Autodesk Fusion 360 part; units mm, degrees
(part 8 of 9)
  line L330 (-42.2083, 57.2942) -> (-37.8782, 54.7942)
  line L331 (-37.8782, 54.7942) -> (-33.5481, 57.2942)
  line L332 (-33.5481, 57.2942) -> (-33.5481, 62.2942)
  line L333 (-33.5481, 62.2942) -> (-37.8782, 64.7942)
  line L334 (-27.718, 64.7942) -> (-32.0481, 62.2942)
  line L335 (-32.0481, 62.2942) -> (-32.0481, 57.2942)
  line L336 (-32.0481, 57.2942) -> (-27.718, 54.7942)
  line L337 (-27.718, 54.7942) -> (-23.3878, 57.2942)
  line L338 (-23.3878, 57.2942) -> (-23.3878, 62.2942)
  line L339 (-23.3878, 62.2942) -> (-27.718, 64.7942)
  line L340 (-17.5577, 64.7942) -> (-21.8878, 62.2942)
  line L341 (-21.8878, 62.2942) -> (-21.8878, 57.2942)
  line L342 (-21.8878, 57.2942) -> (-17.5577, 54.7942)
  line L343 (-17.5577, 54.7942) -> (-13.2276, 57.2942)
  line L344 (-13.2276, 57.2942) -> (-13.2276, 62.2942)
  line L345 (-13.2276, 62.2942) -> (-17.5577, 64.7942)
  line L346 (-103.9199, 73.5933) -> (-108.25, 71.0933)
  line L347 (-108.25, 71.0933) -> (-108.25, 66.0933)
  line L348 (-108.25, 66.0933) -> (-103.9199, 63.5933)
  line L349 (-103.9199, 63.5933) -> (-99.5897, 66.0933)
  line L350 (-99.5897, 66.0933) -> (-99.5897, 71.0933)
  line L351 (-99.5897, 71.0933) -> (-103.9199, 73.5933)
  line L352 (-93.7596, 73.5933) -> (-98.0897, 71.0933)
  line L353 (-98.0897, 71.0933) -> (-98.0897, 66.0933)
  line L354 (-98.0897, 66.0933) -> (-93.7596, 63.5933)
  line L355 (-93.7596, 63.5933) -> (-89.4295, 66.0933)
  line L356 (-89.4295, 66.0933) -> (-89.4295, 71.0933)
  line L357 (-89.4295, 71.0933) -> (-93.7596, 73.5933)
  line L358 (-83.5994, 73.5933) -> (-87.9295, 71.0933)
  line L359 (-87.9295, 71.0933) -> (-87.9295, 66.0933)
  line L360 (-87.9295, 66.0933) -> (-83.5994, 63.5933)
  line L361 (-83.5994, 63.5933) -> (-79.2692, 66.0933)
  line L362 (-79.2692, 66.0933) -> (-79.2692, 71.0933)
  line L363 (-79.2692, 71.0933) -> (-83.5994, 73.5933)
  line L364 (-73.4391, 73.5933) -> (-77.7692, 71.0933)
  line L365 (-77.7692, 71.0933) -> (-77.7692, 66.0933)
  line L366 (-77.7692, 66.0933) -> (-73.4391, 63.5933)
  line L367 (-73.4391, 63.5933) -> (-69.109, 66.0933)
  line L368 (-69.109, 66.0933) -> (-69.109, 71.0933)
  line L369 (-69.109, 71.0933) -> (-73.4391, 73.5933)
  line L370 (-63.2789, 73.5933) -> (-67.609, 71.0933)
  line L371 (-67.609, 71.0933) -> (-67.609, 66.0933)
  line L372 (-67.609, 66.0933) -> (-63.2789, 63.5933)
  line L373 (-63.2789, 63.5933) -> (-58.9487, 66.0933)
  line L374 (-58.9487, 66.0933) -> (-58.9487, 71.0933)
  line L375 (-58.9487, 71.0933) -> (-63.2789, 73.5933)
  line L376 (-53.1186, 73.5933) -> (-57.4487, 71.0933)
  line L377 (-57.4487, 71.0933) -> (-57.4487, 66.0933)
  line L378 (-57.4487, 66.0933) -> (-53.1186, 63.5933)
  line L379 (-53.1186, 63.5933) -> (-48.7885, 66.0933)
  line L380 (-48.7885, 66.0933) -> (-48.7885, 71.0933)
  line L381 (-48.7885, 71.0933) -> (-53.1186, 73.5933)
  line L382 (-42.9583, 73.5933) -> (-47.2885, 71.0933)
  line L383 (-47.2885, 71.0933) -> (-47.2885, 66.0933)
  line L384 (-47.2885, 66.0933) -> (-42.9583, 63.5933)
  line L385 (-42.9583, 63.5933) -> (-38.6282, 66.0933)
  line L386 (-38.6282, 66.0933) -> (-38.6282, 71.0933)
  line L387 (-38.6282, 71.0933) -> (-42.9583, 73.5933)
  line L388 (-32.7981, 73.5933) -> (-37.1282, 71.0933)
  line L389 (-37.1282, 71.0933) -> (-37.1282, 66.0933)
  line L390 (-37.1282, 66.0933) -> (-32.7981, 63.5933)
  line L391 (-32.7981, 63.5933) -> (-28.468, 66.0933)
  line L392 (-28.468, 66.0933) -> (-28.468, 71.0933)
  line L393 (-28.468, 71.0933) -> (-32.7981, 73.5933)
  line L394 (-22.6378, 73.5933) -> (-26.968, 71.0933)
  line L395 (-26.968, 71.0933) -> (-26.968, 66.0933)
  line L396 (-26.968, 66.0933) -> (-22.6378, 63.5933)
  line L397 (-22.6378, 63.5933) -> (-18.3077, 66.0933)
  line L398 (-18.3077, 66.0933) -> (-18.3077, 71.0933)
  line L399 (-18.3077, 71.0933) -> (-22.6378, 73.5933)
  line L400 (-109, 82.3923) -> (-113.3301, 79.8923)
  line L401 (-113.3301, 79.8923) -> (-113.3301, 74.8923)
  line L402 (-113.3301, 74.8923) -> (-109, 72.3923)
  line L403 (-109, 72.3923) -> (-104.6699, 74.8923)
  line L404 (-104.6699, 74.8923) -> (-104.6699, 79.8923)
  line L405 (-104.6699, 79.8923) -> (-109, 82.3923)
  line L406 (-98.8397, 82.3923) -> (-103.1699, 79.8923)
  line L407 (-103.1699, 79.8923) -> (-103.1699, 74.8923)
  line L408 (-103.1699, 74.8923) -> (-98.8397, 72.3923)
  line L409 (-98.8397, 72.3923) -> (-94.5096, 74.8923)
  line L410 (-94.5096, 74.8923) -> (-94.5096, 79.8923)
  line L411 (-94.5096, 79.8923) -> (-98.8397, 82.3923)
  line L412 (-88.6795, 82.3923) -> (-93.0096, 79.8923)
  line L413 (-93.0096, 79.8923) -> (-93.0096, 74.8923)
  line L414 (-93.0096, 74.8923) -> (-88.6795, 72.3923)
  line L415 (-88.6795, 72.3923) -> (-84.3494, 74.8923)
  line L416 (-84.3494, 74.8923) -> (-84.3494, 79.8923)
  line L417 (-84.3494, 79.8923) -> (-88.6795, 82.3923)
  line L418 (-78.5192, 82.3923) -> (-82.8494, 79.8923)
  line L419 (-82.8494, 79.8923) -> (-82.8494, 74.8923)
  line L420 (-82.8494, 74.8923) -> (-78.5192, 72.3923)
  line L421 (-78.5192, 72.3923) -> (-74.1891, 74.8923)
  line L422 (-74.1891, 74.8923) -> (-74.1891, 79.8923)
  line L423 (-74.1891, 79.8923) -> (-78.5192, 82.3923)
  line L424 (-68.359, 82.3923) -> (-72.6891, 79.8923)
  line L425 (-72.6891, 79.8923) -> (-72.6891, 74.8923)
  line L426 (-72.6891, 74.8923) -> (-68.359, 72.3923)
  line L427 (-68.359, 72.3923) -> (-64.0289, 74.8923)
  line L428 (-64.0289, 74.8923) -> (-64.0289, 79.8923)
  line L429 (-64.0289, 79.8923) -> (-68.359, 82.3923)
  line L430 (-58.1987, 82.3923) -> (-62.5289, 79.8923)
  line L431 (-62.5289, 79.8923) -> (-62.5289, 74.8923)
  line L432 (-62.5289, 74.8923) -> (-58.1987, 72.3923)
  line L433 (-58.1987, 72.3923) -> (-53.8686, 74.8923)
  line L434 (-53.8686, 74.8923) -> (-53.8686, 79.8923)
  line L435 (-53.8686, 79.8923) -> (-58.1987, 82.3923)
  line L436 (-48.0385, 82.3923) -> (-52.3686, 79.8923)
  line L437 (-52.3686, 79.8923) -> (-52.3686, 74.8923)
  line L438 (-52.3686, 74.8923) -> (-48.0385, 72.3923)
  line L439 (-48.0385, 72.3923) -> (-43.7083, 74.8923)
  line L440 (-43.7083, 74.8923) -> (-43.7083, 79.8923)
  line L441 (-43.7083, 79.8923) -> (-48.0385, 82.3923)
  line L442 (-37.8782, 82.3923) -> (-42.2083, 79.8923)
  line L443 (-42.2083, 79.8923) -> (-42.2083, 74.8923)
  line L444 (-42.2083, 74.8923) -> (-37.8782, 72.3923)
  line L445 (-37.8782, 72.3923) -> (-33.5481, 74.8923)
  line L446 (-33.5481, 74.8923) -> (-33.5481, 79.8923)
  line L447 (-33.5481, 79.8923) -> (-37.8782, 82.3923)
  line L448 (-27.718, 82.3923) -> (-32.0481, 79.8923)
  line L449 (-32.0481, 79.8923) -> (-32.0481, 74.8923)
  line L450 (-32.0481, 74.8923) -> (-27.718, 72.3923)
  line L451 (-27.718, 72.3923) -> (-23.3878, 74.8923)
  line L452 (-23.3878, 74.8923) -> (-23.3878, 79.8923)
  line L453 (-23.3878, 79.8923) -> (-27.718, 82.3923)
  line L454 (-17.5577, 82.3923) -> (-21.8878, 79.8923)
  line L455 (-21.8878, 79.8923) -> (-21.8878, 74.8923)
  line L456 (-21.8878, 74.8923) -> (-17.5577, 72.3923)
  line L457 (-17.5577, 72.3923) -> (-13.2276, 74.8923)
  line L458 (-13.2276, 74.8923) -> (-13.2276, 79.8923)
  line L459 (-13.2276, 79.8923) -> (-17.5577, 82.3923)
  line L460 (-103.9199, 91.1913) -> (-108.25, 88.6913)
  line L461 (-108.25, 88.6913) -> (-108.25, 83.6913)
  line L462 (-108.25, 83.6913) -> (-103.9199, 81.1913)
  line L463 (-103.9199, 81.1913) -> (-99.5897, 83.6913)
  line L464 (-99.5897, 83.6913) -> (-99.5897, 88.6913)
  line L465 (-99.5897, 88.6913) -> (-103.9199, 91.1913)
  line L466 (-93.7596, 91.1913) -> (-98.0897, 88.6913)
  line L467 (-98.0897, 88.6913) -> (-98.0897, 83.6913)
  line L468 (-98.0897, 83.6913) -> (-93.7596, 81.1913)
  line L469 (-93.7596, 81.1913) -> (-89.4295, 83.6913)
  line L470 (-89.4295, 83.6913) -> (-89.4295, 88.6913)
  line L471 (-89.4295, 88.6913) -> (-93.7596, 91.1913)
  line L472 (-83.5994, 91.1913) -> (-87.9295, 88.6913)
  line L473 (-87.9295, 88.6913) -> (-87.9295, 83.6913)
  line L474 (-87.9295, 83.6913) -> (-83.5994, 81.1913)
  line L475 (-83.5994, 81.1913) -> (-79.2692, 83.6913)
  line L476 (-79.2692, 83.6913) -> (-79.2692, 88.6913)
  line L477 (-79.2692, 88.6913) -> (-83.5994, 91.1913)
  line L478 (-73.4391, 91.1913) -> (-77.7692, 88.6913)
  line L479 (-77.7692, 88.6913) -> (-77.7692, 83.6913)
  line L480 (-77.7692, 83.6913) -> (-73.4391, 81.1913)
  line L481 (-73.4391, 81.1913) -> (-69.109, 83.6913)
  line L482 (-69.109, 83.6913) -> (-69.109, 88.6913)
  line L483 (-69.109, 88.6913) -> (-73.4391, 91.1913)
  line L484 (-63.2789, 91.1913) -> (-67.609, 88.6913)
  line L485 (-67.609, 88.6913) -> (-67.609, 83.6913)
  line L486 (-67.609, 83.6913) -> (-63.2789, 81.1913)
  line L487 (-63.2789, 81.1913) -> (-58.9487, 83.6913)
  line L488 (-58.9487, 83.6913) -> (-58.9487, 88.6913)
  line L489 (-58.9487, 88.6913) -> (-63.2789, 91.1913)
  line L490 (-53.1186, 91.1913) -> (-57.4487, 88.6913)
  line L491 (-57.4487, 88.6913) -> (-57.4487, 83.6913)
  line L492 (-57.4487, 83.6913) -> (-53.1186, 81.1913)
  line L493 (-53.1186, 81.1913) -> (-48.7885, 83.6913)
  line L494 (-48.7885, 83.6913) -> (-48.7885, 88.6913)
  line L495 (-48.7885, 88.6913) -> (-53.1186, 91.1913)
  line L496 (-42.9583, 91.1913) -> (-47.2885, 88.6913)
  line L497 (-47.2885, 88.6913) -> (-47.2885, 83.6913)
  line L498 (-47.2885, 83.6913) -> (-42.9583, 81.1913)
  line L499 (-42.9583, 81.1913) -> (-38.6282, 83.6913)
  line L500 (-38.6282, 83.6913) -> (-38.6282, 88.6913)
  line L501 (-38.6282, 88.6913) -> (-42.9583, 91.1913)
  line L502 (-32.7981, 91.1913) -> (-37.1282, 88.6913)
  line L503 (-37.1282, 88.6913) -> (-37.1282, 83.6913)
  line L504 (-37.1282, 83.6913) -> (-32.7981, 81.1913)
  line L505 (-32.7981, 81.1913) -> (-28.468, 83.6913)
  line L506 (-28.468, 83.6913) -> (-28.468, 88.6913)
  line L507 (-28.468, 88.6913) -> (-32.7981, 91.1913)
  line L508 (-22.6378, 91.1913) -> (-26.968, 88.6913)
  line L509 (-26.968, 88.6913) -> (-26.968, 83.6913)
  line L510 (-26.968, 83.6913) -> (-22.6378, 81.1913)
  line L511 (-22.6378, 81.1913) -> (-18.3077, 83.6913)
  line L512 (-18.3077, 83.6913) -> (-18.3077, 88.6913)
  line L513 (-18.3077, 88.6913) -> (-22.6378, 91.1913)
  line L514 (-109, 99.9904) -> (-113.3301, 97.4904)
  line L515 (-113.3301, 97.4904) -> (-113.3301, 92.4904)
  line L516 (-113.3301, 92.4904) -> (-109, 89.9904)
  line L517 (-109, 89.9904) -> (-104.6699, 92.4904)
  line L518 (-104.6699, 92.4904) -> (-104.6699, 97.4904)
  line L519 (-104.6699, 97.4904) -> (-109, 99.9904)
  line L520 (-98.8397, 99.9904) -> (-103.1699, 97.4904)
  line L521 (-103.1699, 97.4904) -> (-103.1699, 92.4904)
  line L522 (-103.1699, 92.4904) -> (-98.8397, 89.9904)
  line L523 (-98.8397, 89.9904) -> (-94.5096, 92.4904)
  line L524 (-94.5096, 92.4904) -> (-94.5096, 97.4904)
  line L525 (-94.5096, 97.4904) -> (-98.8397, 99.9904)
  line L526 (-88.6795, 99.9904) -> (-93.0096, 97.4904)
  line L527 (-93.0096, 97.4904) -> (-93.0096, 92.4904)
  line L528 (-93.0096, 92.4904) -> (-88.6795, 89.9904)
  line L529 (-88.6795, 89.9904) -> (-84.3494, 92.4904)
  line L530 (-84.3494, 92.4904) -> (-84.3494, 97.4904)
  line L531 (-84.3494, 97.4904) -> (-88.6795, 99.9904)
  line L532 (-78.5192, 99.9904) -> (-82.8494, 97.4904)
  line L533 (-82.8494, 97.4904) -> (-82.8494, 92.4904)
  line L534 (-82.8494, 92.4904) -> (-78.5192, 89.9904)
  line L535 (-78.5192, 89.9904) -> (-74.1891, 92.4904)
  line L536 (-74.1891, 92.4904) -> (-74.1891, 97.4904)
  line L537 (-74.1891, 97.4904) -> (-78.5192, 99.9904)
  line L538 (-68.359, 99.9904) -> (-72.6891, 97.4904)
  line L539 (-72.6891, 97.4904) -> (-72.6891, 92.4904)
  line L540 (-72.6891, 92.4904) -> (-68.359, 89.9904)
  line L541 (-68.359, 89.9904) -> (-64.0289, 92.4904)
  line L542 (-64.0289, 92.4904) -> (-64.0289, 97.4904)
  line L543 (-64.0289, 97.4904) -> (-68.359, 99.9904)
  line L544 (-58.1987, 99.9904) -> (-62.5289, 97.4904)
  line L545 (-62.5289, 97.4904) -> (-62.5289, 92.4904)
  line L546 (-62.5289, 92.4904) -> (-58.1987, 89.9904)
  line L547 (-58.1987, 89.9904) -> (-53.8686, 92.4904)
  line L548 (-53.8686, 92.4904) -> (-53.8686, 97.4904)
  line L549 (-53.8686, 97.4904) -> (-58.1987, 99.9904)
  line L550 (-48.0385, 99.9904) -> (-52.3686, 97.4904)
  line L551 (-52.3686, 97.4904) -> (-52.3686, 92.4904)
  line L552 (-52.3686, 92.4904) -> (-48.0385, 89.9904)
  line L553 (-48.0385, 89.9904) -> (-43.7083, 92.4904)
  line L554 (-43.7083, 92.4904) -> (-43.7083, 97.4904)
  line L555 (-43.7083, 97.4904) -> (-48.0385, 99.9904)
  line L556 (-37.8782, 99.9904) -> (-42.2083, 97.4904)
  line L557 (-42.2083, 97.4904) -> (-42.2083, 92.4904)
  line L558 (-42.2083, 92.4904) -> (-37.8782, 89.9904)
  line L559 (-37.8782, 89.9904) -> (-33.5481, 92.4904)
  line L560 (-33.5481, 92.4904) -> (-33.5481, 97.4904)
  line L561 (-33.5481, 97.4904) -> (-37.8782, 99.9904)
  line L562 (-27.718, 99.9904) -> (-32.0481, 97.4904)
  line L563 (-32.0481, 97.4904) -> (-32.0481, 92.4904)
  line L564 (-32.0481, 92.4904) -> (-27.718, 89.9904)
  line L565 (-27.718, 89.9904) -> (-23.3878, 92.4904)
  line L566 (-23.3878, 92.4904) -> (-23.3878, 97.4904)
  line L567 (-23.3878, 97.4904) -> (-27.718, 99.9904)
  line L568 (-17.5577, 99.9904) -> (-21.8878, 97.4904)
  line L569 (-21.8878, 97.4904) -> (-21.8878, 92.4904)
  line L570 (-21.8878, 92.4904) -> (-17.5577, 89.9904)
  line L571 (-17.5577, 89.9904) -> (-13.2276, 92.4904)
  line L572 (-13.2276, 92.4904) -> (-13.2276, 97.4904)
  line L573 (-13.2276, 97.4904) -> (-17.5577, 99.9904)
  line L574 (-103.9199, 108.7894) -> (-108.25, 106.2894)
  line L575 (-108.25, 106.2894) -> (-108.25, 101.2894)
  line L576 (-108.25, 101.2894) -> (-103.9199, 98.7894)
  line L577 (-103.9199, 98.7894) -> (-99.5897, 101.2894)
  line L578 (-99.5897, 101.2894) -> (-99.5897, 106.2894)
  line L579 (-99.5897, 106.2894) -> (-103.9199, 108.7894)
  line L580 (-93.7596, 108.7894) -> (-98.0897, 106.2894)
  line L581 (-98.0897, 106.2894) -> (-98.0897, 101.2894)
  line L582 (-98.0897, 101.2894) -> (-93.7596, 98.7894)
  line L583 (-93.7596, 98.7894) -> (-89.4295, 101.2894)
  line L584 (-89.4295, 101.2894) -> (-89.4295, 106.2894)
  line L585 (-89.4295, 106.2894) -> (-93.7596, 108.7894)
  line L586 (-83.5994, 108.7894) -> (-87.9295, 106.2894)
  line L587 (-87.9295, 106.2894) -> (-87.9295, 101.2894)
  line L588 (-87.9295, 101.2894) -> (-83.5994, 98.7894)
  line L589 (-83.5994, 98.7894) -> (-79.2692, 101.2894)
  line L590 (-79.2692, 101.2894) -> (-79.2692, 106.2894)
  line L591 (-79.2692, 106.2894) -> (-83.5994, 108.7894)
  line L592 (-73.4391, 108.7894) -> (-77.7692, 106.2894)
  line L593 (-77.7692, 106.2894) -> (-77.7692, 101.2894)
  line L594 (-77.7692, 101.2894) -> (-73.4391, 98.7894)
  line L595 (-73.4391, 98.7894) -> (-69.109, 101.2894)
  line L596 (-69.109, 101.2894) -> (-69.109, 106.2894)
  line L597 (-69.109, 106.2894) -> (-73.4391, 108.7894)
  line L598 (-63.2789, 108.7894) -> (-67.609, 106.2894)
  line L599 (-67.609, 106.2894) -> (-67.609, 101.2894)
  line L600 (-67.609, 101.2894) -> (-63.2789, 98.7894)
  line L601 (-63.2789, 98.7894) -> (-58.9487, 101.2894)
  line L602 (-58.9487, 101.2894) -> (-58.9487, 106.2894)
  line L603 (-58.9487, 106.2894) -> (-63.2789, 108.7894)
  line L604 (-53.1186, 108.7894) -> (-57.4487, 106.2894)
  line L605 (-57.4487, 106.2894) -> (-57.4487, 101.2894)
  line L606 (-57.4487, 101.2894) -> (-53.1186, 98.7894)
  line L607 (-53.1186, 98.7894) -> (-48.7885, 101.2894)
  line L608 (-48.7885, 101.2894) -> (-48.7885, 106.2894)
  line L609 (-48.7885, 106.2894) -> (-53.1186, 108.7894)
  line L610 (-42.9583, 108.7894) -> (-47.2885, 106.2894)
  line L611 (-47.2885, 106.2894) -> (-47.2885, 101.2894)
  line L612 (-47.2885, 101.2894) -> (-42.9583, 98.7894)
  line L613 (-42.9583, 98.7894) -> (-38.6282, 101.2894)
  line L614 (-38.6282, 101.2894) -> (-38.6282, 106.2894)
  line L615 (-38.6282, 106.2894) -> (-42.9583, 108.7894)
  line L616 (-32.7981, 108.7894) -> (-37.1282, 106.2894)
  line L617 (-37.1282, 106.2894) -> (-37.1282, 101.2894)
  line L618 (-37.1282, 101.2894) -> (-32.7981, 98.7894)
  line L619 (-32.7981, 98.7894) -> (-28.468, 101.2894)
  line L620 (-28.468, 101.2894) -> (-28.468, 106.2894)
  line L621 (-28.468, 106.2894) -> (-32.7981, 108.7894)
  line L622 (-22.6378, 108.7894) -> (-26.968, 106.2894)
  line L623 (-26.968, 106.2894) -> (-26.968, 101.2894)
  line L624 (-26.968, 101.2894) -> (-22.6378, 98.7894)
  line L625 (-22.6378, 98.7894) -> (-18.3077, 101.2894)
  line L626 (-18.3077, 101.2894) -> (-18.3077, 106.2894)
  line L627 (-18.3077, 106.2894) -> (-22.6378, 108.7894)
  line L628 (-109, 117.5885) -> (-113.3301, 115.0885)
  line L629 (-113.3301, 115.0885) -> (-113.3301, 110.0885)
  line L630 (-113.3301, 110.0885) -> (-109, 107.5885)
  line L631 (-109, 107.5885) -> (-104.6699, 110.0885)
  line L632 (-104.6699, 110.0885) -> (-104.6699, 115.0885)
  line L633 (-104.6699, 115.0885) -> (-109, 117.5885)
  line L634 (-98.8397, 117.5885) -> (-103.1699, 115.0885)
  line L635 (-103.1699, 115.0885) -> (-103.1699, 110.0885)
  line L636 (-103.1699, 110.0885) -> (-98.8397, 107.5885)
  line L637 (-98.8397, 107.5885) -> (-94.5096, 110.0885)
  line L638 (-94.5096, 110.0885) -> (-94.5096, 115.0885)
  line L639 (-94.5096, 115.0885) -> (-98.8397, 117.5885)
  line L640 (-88.6795, 117.5885) -> (-93.0096, 115.0885)
  line L641 (-93.0096, 115.0885) -> (-93.0096, 110.0885)
  line L642 (-93.0096, 110.0885) -> (-88.6795, 107.5885)
  line L643 (-88.6795, 107.5885) -> (-84.3494, 110.0885)
  line L644 (-84.3494, 110.0885) -> (-84.3494, 115.0885)
  line L645 (-84.3494, 115.0885) -> (-88.6795, 117.5885)
  line L646 (-78.5192, 117.5885) -> (-82.8494, 115.0885)
  line L647 (-82.8494, 115.0885) -> (-82.8494, 110.0885)
  line L648 (-82.8494, 110.0885) -> (-78.5192, 107.5885)
  line L649 (-78.5192, 107.5885) -> (-74.1891, 110.0885)
  line L650 (-74.1891, 110.0885) -> (-74.1891, 115.0885)
  line L651 (-74.1891, 115.0885) -> (-78.5192, 117.5885)
  line L652 (-68.359, 117.5885) -> (-72.6891, 115.0885)
  line L653 (-72.6891, 115.0885) -> (-72.6891, 110.0885)
  line L654 (-72.6891, 110.0885) -> (-68.359, 107.5885)
  line L655 (-68.359, 107.5885) -> (-64.0289, 110.0885)
  line L656 (-64.0289, 110.0885) -> (-64.0289, 115.0885)
  line L657 (-64.0289, 115.0885) -> (-68.359, 117.5885)
  line L658 (-58.1987, 117.5885) -> (-62.5289, 115.0885)
  line L659 (-62.5289, 115.0885) -> (-62.5289, 110.0885)
  line L660 (-62.5289, 110.0885) -> (-58.1987, 107.5885)
  line L661 (-58.1987, 107.5885) -> (-53.8686, 110.0885)
  line L662 (-53.8686, 110.0885) -> (-53.8686, 115.0885)
  line L663 (-53.8686, 115.0885) -> (-58.1987, 117.5885)
  line L664 (-48.0385, 117.5885) -> (-52.3686, 115.0885)
  line L665 (-52.3686, 115.0885) -> (-52.3686, 110.0885)
  line L666 (-52.3686, 110.0885) -> (-48.0385, 107.5885)
  line L667 (-48.0385, 107.5885) -> (-43.7083, 110.0885)
  line L668 (-43.7083, 110.0885) -> (-43.7083, 115.0885)
  line L669 (-43.7083, 115.0885) -> (-48.0385, 117.5885)
  line L670 (-37.8782, 117.5885) -> (-42.2083, 115.0885)
  line L671 (-42.2083, 115.0885) -> (-42.2083, 110.0885)
  line L672 (-42.2083, 110.0885) -> (-37.8782, 107.5885)
  line L673 (-37.8782, 107.5885) -> (-33.5481, 110.0885)
  line L674 (-33.5481, 110.0885) -> (-33.5481, 115.0885)
  line L675 (-33.5481, 115.0885) -> (-37.8782, 117.5885)
  line L676 (-27.718, 117.5885) -> (-32.0481, 115.0885)
  line L677 (-32.0481, 115.0885) -> (-32.0481, 110.0885)
  line L678 (-32.0481, 110.0885) -> (-27.718, 107.5885)
  line L679 (-27.718, 107.5885) -> (-23.3878, 110.0885)
  line L680 (-23.3878, 110.0885) -> (-23.3878, 115.0885)
  line L681 (-23.3878, 115.0885) -> (-27.718, 117.5885)
  line L682 (-17.5577, 117.5885) -> (-21.8878, 115.0885)
  line L683 (-21.8878, 115.0885) -> (-21.8878, 110.0885)
  line L684 (-21.8878, 110.0885) -> (-17.5577, 107.5885)
  line L685 (-17.5577, 107.5885) -> (-13.2276, 110.0885)
  line L686 (-13.2276, 110.0885) -> (-13.2276, 115.0885)
  line L687 (-13.2276, 115.0885) -> (-17.5577, 117.5885)
extrude "拉伸26" cut sketch "草图26" against normal blind 5 contours L4 L5 L6 L7 L8 L9 | L10 L11 L12 L13 L14 L15 | L16 L17 L18 L19 L20 L21 | L22 L23 L24 L25 L26 L27 | L28 L29 L30 L31 L32 L33 | L34 L35 L36 L37 L38 L39 | L40 L41 L42 L43 L44 L45 | L46 L47 L48 L49 L50 L51 | L52 L53 L54 L55 L56 L57 | L58 L59 L60 L61 L62 L63 | L64 L65 L66 L67 L68 L69 | L70 L71 L72 L73 L74 L75 | L76 L77 L78 L79 L80 L81 | L82 L83 L84 L85 L86 L87 | L88 L89 L90 L91 L92 L93 | L94 L95 L96 L97 L98 L99 | L100 L101 L102 L103 L104 L105 | L106 L107 L108 L109 L110 L111 | L112 L113 L114 L115 L116 L117 | L118 L119 L120 L121 L122 L123 | L124 L125 L126 L127 L128 L129 | L130 L131 L132 L133 L134 L135 | L136 L137 L138 L139 L140 L141 | L142 L143 L144 L145 L146 L147 | L148 L149 L150 L151 L152 L153 | L154 L155 L156 L157 L158 L159 | L160 L161 L162 L163 L164 L165 | L166 L167 L168 L169 L170 L171 | L172 L173 L174 L175 L176 L177 | L178 L179 L180 L181 L182 L183 | L184 L185 L186 L187 L188 L189 | L190 L191 L192 L193 L194 L195 | L196 L197 L198 L199 L200 L201 | L202 L203 L204 L205 L206 L207 | L208 L209 L210 L211 L212 L213 | L214 L215 L216 L217 L218 L219 | L220 L221 L222 L223 L224 L225 | L226 L227 L228 L229 L230 L231 | L232 L233 L234 L235 L236 L237 | L238 L239 L240 L241 L242 L243 | L244 L245 L246 L247 L248 L249 | L250 L251 L252 L253 L254 L255 | L256 L257 L258 L259 L260 L261 | L262 L263 L264 L265 L266 L267 | L268 L269 L270 L271 L272 L273 | L274 L275 L276 L277 L278 L279 | L280 L281 L282 L283 L284 L285 | L286 L287 L288 L289 L290 L291 | L292 L293 L294 L295 L296 L297 | L298 L299 L300 L301 L302 L303 | L304 L305 L306 L307 L308 L309 | L310 L311 L312 L313 L314 L315 | L316 L317 L318 L319 L320 L321 | L322 L323 L324 L325 L326 L327 | L328 L329 L330 L331 L332 L333 | L334 L335 L336 L337 L338 L339 | L340 L341 L342 L343 L344 L345 | L346 L347 L348 L349 L350 L351 | L352 L353 L354 L355 L356 L357 | L358 L359 L360 L361 L362 L363 | L364 L365 L366 L367 L368 L369 | L370 L371 L372 L373 L374 L375 | L376 L377 L378 L379 L380 L381 | L382 L383 L384 L385 L386 L387 | L388 L389 L390 L391 L392 L393 | L394 L395 L396 L397 L398 L399 | L400 L401 L402 L403 L404 L405 | L406 L407 L408 L409 L410 L411 | L412 L413 L414 L415 L416 L417 | L418 L419 L420 L421 L422 L423 | L424 L425 L426 L427 L428 L429 | L430 L431 L432 L433 L434 L435 | L436 L437 L438 L439 L440 L441 | L442 L443 L444 L445 L446 L447 | L448 L449 L450 L451 L452 L453 | L454 L455 L456 L457 L458 L459 | L460 L461 L462 L463 L464 L465 | L466 L467 L468 L469 L470 L471 | L472 L473 L474 L475 L476 L477 | L478 L479 L480 L481 L482 L483 | L484 L485 L486 L487 L488 L489 | L490 L491 L492 L493 L494 L495 | L496 L497 L498 L499 L500 L501 | L502 L503 L504 L505 L506 L507 | L508 L509 L510 L511 L512 L513 | L514 L515 L516 L517 L518 L519 | L520 L521 L522 L523 L524 L525 | L526 L527 L528 L529 L530 L531 | L532 L533 L534 L535 L536 L537 | L538 L539 L540 L541 L542 L543 | L544 L545 L546 L547 L548 L549 | L550 L551 L552 L553 L554 L555 | L556 L557 L558 L559 L560 L561 | L562 L563 L564 L565 L566 L567 | L568 L569 L570 L571 L572 L573 | L574 L575 L576 L577 L578 L579 | L580 L581 L582 L583 L584 L585 | L586 L587 L588 L589 L590 L591 | L592 L593 L594 L595 L596 L597 | L598 L599 L600 L601 L602 L603 | L604 L605 L606 L607 L608 L609 | L610 L611 L612 L613 L614 L615 | L616 L617 L618 L619 L620 L621 | L622 L623 L624 L625 L626 L627 | L628 L629 L630 L631 L632 L633 | L634 L635 L636 L637 L638 L639 | L640 L641 L642 L643 L644 L645 | L646 L647 L648 L649 L650 L651 | L652 L653 L654 L655 L656 L657 | L658 L659 L660 L661 L662 L663 | L664 L665 L666 L667 L668 L669 | L670 L671 L672 L673 L674 L675 | L676 L677 L678 L679 L680 L681 | L682 L683 L684 L685 L686 L687 bodies 1 4
sketch "草图27" plane through (116, 0, 0) normal (-1, 0, 0) x (0, -1, 0)
  line L0 (7, 0) -> (116, 0)
  line L1 (116, 0) -> (116, 120)
  line L2 (116, 120) -> (7, 120)
  line L3 (7, 120) -> (7, 0)
  line L4 (19.0801, 20.799) -> (14.75, 18.299)
  line L5 (14.75, 18.299) -> (14.75, 13.299)
  line L6 (14.75, 13.299) -> (19.0801, 10.799)
  line L7 (19.0801, 10.799) -> (23.4103, 13.299)
  line L8 (23.4103, 13.299) -> (23.4103, 18.299)
  line L9 (23.4103, 18.299) -> (19.0801, 20.799)
  line L10 (29.2404, 20.799) -> (24.9103, 18.299)
  line L11 (24.9103, 18.299) -> (24.9103, 13.299)
  line L12 (24.9103, 13.299) -> (29.2404, 10.799)
  line L13 (29.2404, 10.799) -> (33.5705, 13.299)
  line L14 (33.5705, 13.299) -> (33.5705, 18.299)
  line L15 (33.5705, 18.299) -> (29.2404, 20.799)
  line L16 (39.4006, 20.799) -> (35.0705, 18.299)
  line L17 (35.0705, 18.299) -> (35.0705, 13.299)
  line L18 (35.0705, 13.299) -> (39.4006, 10.799)
  line L19 (39.4006, 10.799) -> (43.7308, 13.299)
  line L20 (43.7308, 13.299) -> (43.7308, 18.299)
  line L21 (43.7308, 18.299) -> (39.4006, 20.799)
  line L22 (49.5609, 20.799) -> (45.2308, 18.299)
  line L23 (45.2308, 18.299) -> (45.2308, 13.299)
  line L24 (45.2308, 13.299) -> (49.5609, 10.799)
  line L25 (49.5609, 10.799) -> (53.891, 13.299)
  line L26 (53.891, 13.299) -> (53.891, 18.299)
  line L27 (53.891, 18.299) -> (49.5609, 20.799)
  line L28 (59.7211, 20.799) -> (55.391, 18.299)
  line L29 (55.391, 18.299) -> (55.391, 13.299)
  line L30 (55.391, 13.299) -> (59.7211, 10.799)
  line L31 (59.7211, 10.799) -> (64.0513, 13.299)
  line L32 (64.0513, 13.299) -> (64.0513, 18.299)
  line L33 (64.0513, 18.299) -> (59.7211, 20.799)
  line L34 (69.8814, 20.799) -> (65.5513, 18.299)
  line L35 (65.5513, 18.299) -> (65.5513, 13.299)
  line L36 (65.5513, 13.299) -> (69.8814, 10.799)
  line L37 (69.8814, 10.799) -> (74.2115, 13.299)
  line L38 (74.2115, 13.299) -> (74.2115, 18.299)
  line L39 (74.2115, 18.299) -> (69.8814, 20.799)
  line L40 (80.0416, 20.799) -> (75.7115, 18.299)
  line L41 (75.7115, 18.299) -> (75.7115, 13.299)
  line L42 (75.7115, 13.299) -> (80.0416, 10.799)
  line L43 (80.0416, 10.799) -> (84.3718, 13.299)
  line L44 (84.3718, 13.299) -> (84.3718, 18.299)
  line L45 (84.3718, 18.299) -> (80.0416, 20.799)
  line L46 (90.2019, 20.799) -> (85.8718, 18.299)
  line L47 (85.8718, 18.299) -> (85.8718, 13.299)
  line L48 (85.8718, 13.299) -> (90.2019, 10.799)
  line L49 (90.2019, 10.799) -> (94.532, 13.299)
  line L50 (94.532, 13.299) -> (94.532, 18.299)
  line L51 (94.532, 18.299) -> (90.2019, 20.799)
  line L52 (100.3622, 20.799) -> (96.032, 18.299)
  line L53 (96.032, 18.299) -> (96.032, 13.299)
  line L54 (96.032, 13.299) -> (100.3622, 10.799)
  line L55 (100.3622, 10.799) -> (104.6923, 13.299)
  line L56 (104.6923, 13.299) -> (104.6923, 18.299)
  line L57 (104.6923, 18.299) -> (100.3622, 20.799)
  line L58 (14, 29.5981) -> (9.6699, 27.0981)
  line L59 (9.6699, 27.0981) -> (9.6699, 22.0981)
  line L60 (9.6699, 22.0981) -> (14, 19.5981)
  line L61 (14, 19.5981) -> (18.3301, 22.0981)
  line L62 (18.3301, 22.0981) -> (18.3301, 27.0981)
  line L63 (18.3301, 27.0981) -> (14, 29.5981)
  line L64 (24.1603, 29.5981) -> (19.8301, 27.0981)
  line L65 (19.8301, 27.0981) -> (19.8301, 22.0981)
  line L66 (19.8301, 22.0981) -> (24.1603, 19.5981)
  line L67 (24.1603, 19.5981) -> (28.4904, 22.0981)
  line L68 (28.4904, 22.0981) -> (28.4904, 27.0981)
  line L69 (28.4904, 27.0981) -> (24.1603, 29.5981)
  line L70 (34.3205, 29.5981) -> (29.9904, 27.0981)
  line L71 (29.9904, 27.0981) -> (29.9904, 22.0981)
  line L72 (29.9904, 22.0981) -> (34.3205, 19.5981)
  line L73 (34.3205, 19.5981) -> (38.6506, 22.0981)
  line L74 (38.6506, 22.0981) -> (38.6506, 27.0981)
  line L75 (38.6506, 27.0981) -> (34.3205, 29.5981)
  line L76 (44.4808, 29.5981) -> (40.1506, 27.0981)
  line L77 (40.1506, 27.0981) -> (40.1506, 22.0981)
  line L78 (40.1506, 22.0981) -> (44.4808, 19.5981)
  line L79 (44.4808, 19.5981) -> (48.8109, 22.0981)
  line L80 (48.8109, 22.0981) -> (48.8109, 27.0981)
  line L81 (48.8109, 27.0981) -> (44.4808, 29.5981)
  line L82 (54.641, 29.5981) -> (50.3109, 27.0981)
  line L83 (50.3109, 27.0981) -> (50.3109, 22.0981)
  line L84 (50.3109, 22.0981) -> (54.641, 19.5981)
  line L85 (54.641, 19.5981) -> (58.9711, 22.0981)
  line L86 (58.9711, 22.0981) -> (58.9711, 27.0981)
  line L87 (58.9711, 27.0981) -> (54.641, 29.5981)
  line L88 (64.8013, 29.5981) -> (60.4711, 27.0981)
  line L89 (60.4711, 27.0981) -> (60.4711, 22.0981)
  line L90 (60.4711, 22.0981) -> (64.8013, 19.5981)
  line L91 (64.8013, 19.5981) -> (69.1314, 22.0981)
  line L92 (69.1314, 22.0981) -> (69.1314, 27.0981)
  line L93 (69.1314, 27.0981) -> (64.8013, 29.5981)
  line L94 (74.9615, 29.5981) -> (70.6314, 27.0981)
  line L95 (70.6314, 27.0981) -> (70.6314, 22.0981)
  line L96 (70.6314, 22.0981) -> (74.9615, 19.5981)
  line L97 (74.9615, 19.5981) -> (79.2916, 22.0981)
  line L98 (79.2916, 22.0981) -> (79.2916, 27.0981)
  line L99 (79.2916, 27.0981) -> (74.9615, 29.5981)
  line L100 (85.1218, 29.5981) -> (80.7916, 27.0981)
  line L101 (80.7916, 27.0981) -> (80.7916, 22.0981)
  line L102 (80.7916, 22.0981) -> (85.1218, 19.5981)
  line L103 (85.1218, 19.5981) -> (89.4519, 22.0981)
  line L104 (89.4519, 22.0981) -> (89.4519, 27.0981)
  line L105 (89.4519, 27.0981) -> (85.1218, 29.5981)
  line L106 (95.282, 29.5981) -> (90.9519, 27.0981)
  line L107 (90.9519, 27.0981) -> (90.9519, 22.0981)
  line L108 (90.9519, 22.0981) -> (95.282, 19.5981)
  line L109 (95.282, 19.5981) -> (99.6122, 22.0981)
  line L110 (99.6122, 22.0981) -> (99.6122, 27.0981)
  line L111 (99.6122, 27.0981) -> (95.282, 29.5981)
  line L112 (105.4423, 29.5981) -> (101.1122, 27.0981)
  line L113 (101.1122, 27.0981) -> (101.1122, 22.0981)
  line L114 (101.1122, 22.0981) -> (105.4423, 19.5981)
  line L115 (105.4423, 19.5981) -> (109.7724, 22.0981)
  line L116 (109.7724, 22.0981) -> (109.7724, 27.0981)
  line L117 (109.7724, 27.0981) -> (105.4423, 29.5981)
  line L118 (19.0801, 38.3971) -> (14.75, 35.8971)
  line L119 (14.75, 35.8971) -> (14.75, 30.8971)
  line L120 (14.75, 30.8971) -> (19.0801, 28.3971)
  line L121 (19.0801, 28.3971) -> (23.4103, 30.8971)
  line L122 (23.4103, 30.8971) -> (23.4103, 35.8971)
  line L123 (23.4103, 35.8971) -> (19.0801, 38.3971)
  line L124 (29.2404, 38.3971) -> (24.9103, 35.8971)
  line L125 (24.9103, 35.8971) -> (24.9103, 30.8971)
  line L126 (24.9103, 30.8971) -> (29.2404, 28.3971)
  line L127 (29.2404, 28.3971) -> (33.5705, 30.8971)
  line L128 (33.5705, 30.8971) -> (33.5705, 35.8971)
  line L129 (33.5705, 35.8971) -> (29.2404, 38.3971)
  line L130 (39.4006, 38.3971) -> (35.0705, 35.8971)
  line L131 (35.0705, 35.8971) -> (35.0705, 30.8971)
  line L132 (35.0705, 30.8971) -> (39.4006, 28.3971)
  line L133 (39.4006, 28.3971) -> (43.7308, 30.8971)
  line L134 (43.7308, 30.8971) -> (43.7308, 35.8971)
  line L135 (43.7308, 35.8971) -> (39.4006, 38.3971)
  line L136 (49.5609, 38.3971) -> (45.2308, 35.8971)
  line L137 (45.2308, 35.8971) -> (45.2308, 30.8971)
  line L138 (45.2308, 30.8971) -> (49.5609, 28.3971)
  line L139 (49.5609, 28.3971) -> (53.891, 30.8971)
  line L140 (53.891, 30.8971) -> (53.891, 35.8971)
  line L141 (53.891, 35.8971) -> (49.5609, 38.3971)
  line L142 (59.7211, 38.3971) -> (55.391, 35.8971)
  line L143 (55.391, 35.8971) -> (55.391, 30.8971)
  line L144 (55.391, 30.8971) -> (59.7211, 28.3971)
  line L145 (59.7211, 28.3971) -> (64.0513, 30.8971)
  line L146 (64.0513, 30.8971) -> (64.0513, 35.8971)
  line L147 (64.0513, 35.8971) -> (59.7211, 38.3971)
  line L148 (69.8814, 38.3971) -> (65.5513, 35.8971)
  line L149 (65.5513, 35.8971) -> (65.5513, 30.8971)
  line L150 (65.5513, 30.8971) -> (69.8814, 28.3971)
  line L151 (69.8814, 28.3971) -> (74.2115, 30.8971)
  line L152 (74.2115, 30.8971) -> (74.2115, 35.8971)
  line L153 (74.2115, 35.8971) -> (69.8814, 38.3971)
  line L154 (80.0416, 38.3971) -> (75.7115, 35.8971)
  line L155 (75.7115, 35.8971) -> (75.7115, 30.8971)
  line L156 (75.7115, 30.8971) -> (80.0416, 28.3971)
  line L157 (80.0416, 28.3971) -> (84.3718, 30.8971)
  line L158 (84.3718, 30.8971) -> (84.3718, 35.8971)
  line L159 (84.3718, 35.8971) -> (80.0416, 38.3971)
  line L160 (90.2019, 38.3971) -> (85.8718, 35.8971)
  line L161 (85.8718, 35.8971) -> (85.8718, 30.8971)
  line L162 (85.8718, 30.8971) -> (90.2019, 28.3971)
  line L163 (90.2019, 28.3971) -> (94.532, 30.8971)
  line L164 (94.532, 30.8971) -> (94.532, 35.8971)
  line L165 (94.532, 35.8971) -> (90.2019, 38.3971)
  line L166 (100.3622, 38.3971) -> (96.032, 35.8971)
  line L167 (96.032, 35.8971) -> (96.032, 30.8971)
  line L168 (96.032, 30.8971) -> (100.3622, 28.3971)
  line L169 (100.3622, 28.3971) -> (104.6923, 30.8971)
  line L170 (104.6923, 30.8971) -> (104.6923, 35.8971)
  line L171 (104.6923, 35.8971) -> (100.3622, 38.3971)
  line L172 (14, 47.1962) -> (9.6699, 44.6962)
  line L173 (9.6699, 44.6962) -> (9.6699, 39.6962)
  line L174 (9.6699, 39.6962) -> (14, 37.1962)
  line L175 (14, 37.1962) -> (18.3301, 39.6962)
  line L176 (18.3301, 39.6962) -> (18.3301, 44.6962)
  line L177 (18.3301, 44.6962) -> (14, 47.1962)
  line L178 (24.1603, 47.1962) -> (19.8301, 44.6962)
  line L179 (19.8301, 44.6962) -> (19.8301, 39.6962)
  line L180 (19.8301, 39.6962) -> (24.1603, 37.1962)
  line L181 (24.1603, 37.1962) -> (28.4904, 39.6962)
  line L182 (28.4904, 39.6962) -> (28.4904, 44.6962)
  line L183 (28.4904, 44.6962) -> (24.1603, 47.1962)
  line L184 (34.3205, 47.1962) -> (29.9904, 44.6962)
  line L185 (29.9904, 44.6962) -> (29.9904, 39.6962)
  line L186 (29.9904, 39.6962) -> (34.3205, 37.1962)
  line L187 (34.3205, 37.1962) -> (38.6506, 39.6962)
  line L188 (38.6506, 39.6962) -> (38.6506, 44.6962)
  line L189 (38.6506, 44.6962) -> (34.3205, 47.1962)
  line L190 (44.4808, 47.1962) -> (40.1506, 44.6962)
  line L191 (40.1506, 44.6962) -> (40.1506, 39.6962)
  line L192 (40.1506, 39.6962) -> (44.4808, 37.1962)
  line L193 (44.4808, 37.1962) -> (48.8109, 39.6962)
  line L194 (48.8109, 39.6962) -> (48.8109, 44.6962)
  line L195 (48.8109, 44.6962) -> (44.4808, 47.1962)
  line L196 (54.641, 47.1962) -> (50.3109, 44.6962)
  line L197 (50.3109, 44.6962) -> (50.3109, 39.6962)
  line L198 (50.3109, 39.6962) -> (54.641, 37.1962)
  line L199 (54.641, 37.1962) -> (58.9711, 39.6962)
  line L200 (58.9711, 39.6962) -> (58.9711, 44.6962)
  line L201 (58.9711, 44.6962) -> (54.641, 47.1962)
  line L202 (64.8013, 47.1962) -> (60.4711, 44.6962)
  line L203 (60.4711, 44.6962) -> (60.4711, 39.6962)
  line L204 (60.4711, 39.6962) -> (64.8013, 37.1962)
  line L205 (64.8013, 37.1962) -> (69.1314, 39.6962)
  line L206 (69.1314, 39.6962) -> (69.1314, 44.6962)
  line L207 (69.1314, 44.6962) -> (64.8013, 47.1962)
  line L208 (74.9615, 47.1962) -> (70.6314, 44.6962)
  line L209 (70.6314, 44.6962) -> (70.6314, 39.6962)
  line L210 (70.6314, 39.6962) -> (74.9615, 37.1962)
  line L211 (74.9615, 37.1962) -> (79.2916, 39.6962)
  line L212 (79.2916, 39.6962) -> (79.2916, 44.6962)
  line L213 (79.2916, 44.6962) -> (74.9615, 47.1962)
  line L214 (85.1218, 47.1962) -> (80.7916, 44.6962)
  line L215 (80.7916, 44.6962) -> (80.7916, 39.6962)
  line L216 (80.7916, 39.6962) -> (85.1218, 37.1962)
  line L217 (85.1218, 37.1962) -> (89.4519, 39.6962)
  line L218 (89.4519, 39.6962) -> (89.4519, 44.6962)
  line L219 (89.4519, 44.6962) -> (85.1218, 47.1962)
  line L220 (95.282, 47.1962) -> (90.9519, 44.6962)
  line L221 (90.9519, 44.6962) -> (90.9519, 39.6962)
  line L222 (90.9519, 39.6962) -> (95.282, 37.1962)
  line L223 (95.282, 37.1962) -> (99.6122, 39.6962)
  line L224 (99.6122, 39.6962) -> (99.6122, 44.6962)
  line L225 (99.6122, 44.6962) -> (95.282, 47.1962)
  line L226 (105.4423, 47.1962) -> (101.1122, 44.6962)
  line L227 (101.1122, 44.6962) -> (101.1122, 39.6962)
  line L228 (101.1122, 39.6962) -> (105.4423, 37.1962)
  line L229 (105.4423, 37.1962) -> (109.7724, 39.6962)
  line L230 (109.7724, 39.6962) -> (109.7724, 44.6962)
  line L231 (109.7724, 44.6962) -> (105.4423, 47.1962)
  line L232 (19.0801, 55.9952) -> (14.75, 53.4952)
  line L233 (14.75, 53.4952) -> (14.75, 48.4952)
  line L234 (14.75, 48.4952) -> (19.0801, 45.9952)
  line L235 (19.0801, 45.9952) -> (23.4103, 48.4952)
  line L236 (23.4103, 48.4952) -> (23.4103, 53.4952)
  line L237 (23.4103, 53.4952) -> (19.0801, 55.9952)
  line L238 (29.2404, 55.9952) -> (24.9103, 53.4952)
  line L239 (24.9103, 53.4952) -> (24.9103, 48.4952)
  line L240 (24.9103, 48.4952) -> (29.2404, 45.9952)
  line L241 (29.2404, 45.9952) -> (33.5705, 48.4952)
  line L242 (33.5705, 48.4952) -> (33.5705, 53.4952)
  line L243 (33.5705, 53.4952) -> (29.2404, 55.9952)
  line L244 (39.4006, 55.9952) -> (35.0705, 53.4952)
  line L245 (35.0705, 53.4952) -> (35.0705, 48.4952)
  line L246 (35.0705, 48.4952) -> (39.4006, 45.9952)
  line L247 (39.4006, 45.9952) -> (43.7308, 48.4952)
  line L248 (43.7308, 48.4952) -> (43.7308, 53.4952)
  line L249 (43.7308, 53.4952) -> (39.4006, 55.9952)
  line L250 (49.5609, 55.9952) -> (45.2308, 53.4952)
  line L251 (45.2308, 53.4952) -> (45.2308, 48.4952)
  line L252 (45.2308, 48.4952) -> (49.5609, 45.9952)
  line L253 (49.5609, 45.9952) -> (53.891, 48.4952)
  line L254 (53.891, 48.4952) -> (53.891, 53.4952)
  line L255 (53.891, 53.4952) -> (49.5609, 55.9952)
  line L256 (59.7211, 55.9952) -> (55.391, 53.4952)
  line L257 (55.391, 53.4952) -> (55.391, 48.4952)
  line L258 (55.391, 48.4952) -> (59.7211, 45.9952)
  line L259 (59.7211, 45.9952) -> (64.0513, 48.4952)
  line L260 (64.0513, 48.4952) -> (64.0513, 53.4952)
  line L261 (64.0513, 53.4952) -> (59.7211, 55.9952)
  line L262 (69.8814, 55.9952) -> (65.5513, 53.4952)
  line L263 (65.5513, 53.4952) -> (65.5513, 48.4952)
  line L264 (65.5513, 48.4952) -> (69.8814, 45.9952)
  line L265 (69.8814, 45.9952) -> (74.2115, 48.4952)
  line L266 (74.2115, 48.4952) -> (74.2115, 53.4952)
  line L267 (74.2115, 53.4952) -> (69.8814, 55.9952)
  line L268 (80.0416, 55.9952) -> (75.7115, 53.4952)
  line L269 (75.7115, 53.4952) -> (75.7115, 48.4952)
  line L270 (75.7115, 48.4952) -> (80.0416, 45.9952)
  line L271 (80.0416, 45.9952) -> (84.3718, 48.4952)
  line L272 (84.3718, 48.4952) -> (84.3718, 53.4952)
  line L273 (84.3718, 53.4952) -> (80.0416, 55.9952)
  line L274 (90.2019, 55.9952) -> (85.8718, 53.4952)
  line L275 (85.8718, 53.4952) -> (85.8718, 48.4952)
  line L276 (85.8718, 48.4952) -> (90.2019, 45.9952)
  line L277 (90.2019, 45.9952) -> (94.532, 48.4952)
  line L278 (94.532, 48.4952) -> (94.532, 53.4952)
  line L279 (94.532, 53.4952) -> (90.2019, 55.9952)
  line L280 (100.3622, 55.9952) -> (96.032, 53.4952)
  line L281 (96.032, 53.4952) -> (96.032, 48.4952)
  line L282 (96.032, 48.4952) -> (100.3622, 45.9952)
  line L283 (100.3622, 45.9952) -> (104.6923, 48.4952)
  line L284 (104.6923, 48.4952) -> (104.6923, 53.4952)
  line L285 (104.6923, 53.4952) -> (100.3622, 55.9952)
  line L286 (14, 64.7942) -> (9.6699, 62.2942)
  line L287 (9.6699, 62.2942) -> (9.6699, 57.2942)
  line L288 (9.6699, 57.2942) -> (14, 54.7942)
  line L289 (14, 54.7942) -> (18.3301, 57.2942)
  line L290 (18.3301, 57.2942) -> (18.3301, 62.2942)
  line L291 (18.3301, 62.2942) -> (14, 64.7942)
  line L292 (24.1603, 64.7942) -> (19.8301, 62.2942)
  line L293 (19.8301, 62.2942) -> (19.8301, 57.2942)
  line L294 (19.8301, 57.2942) -> (24.1603, 54.7942)
  line L295 (24.1603, 54.7942) -> (28.4904, 57.2942)
  line L296 (28.4904, 57.2942) -> (28.4904, 62.2942)
  line L297 (28.4904, 62.2942) -> (24.1603, 64.7942)
  line L298 (34.3205, 64.7942) -> (29.9904, 62.2942)
  line L299 (29.9904, 62.2942) -> (29.9904, 57.2942)
  line L300 (29.9904, 57.2942) -> (34.3205, 54.7942)
  line L301 (34.3205, 54.7942) -> (38.6506, 57.2942)
  line L302 (38.6506, 57.2942) -> (38.6506, 62.2942)
  line L303 (38.6506, 62.2942) -> (34.3205, 64.7942)
  line L304 (44.4808, 64.7942) -> (40.1506, 62.2942)
  line L305 (40.1506, 62.2942) -> (40.1506, 57.2942)
  line L306 (40.1506, 57.2942) -> (44.4808, 54.7942)
  line L307 (44.4808, 54.7942) -> (48.8109, 57.2942)
  line L308 (48.8109, 57.2942) -> (48.8109, 62.2942)
  line L309 (48.8109, 62.2942) -> (44.4808, 64.7942)
  line L310 (54.641, 64.7942) -> (50.3109, 62.2942)
  line L311 (50.3109, 62.2942) -> (50.3109, 57.2942)
  line L312 (50.3109, 57.2942) -> (54.641, 54.7942)
  line L313 (54.641, 54.7942) -> (58.9711, 57.2942)
  line L314 (58.9711, 57.2942) -> (58.9711, 62.2942)
  line L315 (58.9711, 62.2942) -> (54.641, 64.7942)
  line L316 (64.8013, 64.7942) -> (60.4711, 62.2942)
  line L317 (60.4711, 62.2942) -> (60.4711, 57.2942)
  line L318 (60.4711, 57.2942) -> (64.8013, 54.7942)
  line L319 (64.8013, 54.7942) -> (69.1314, 57.2942)
  line L320 (69.1314, 57.2942) -> (69.1314, 62.2942)
  line L321 (69.1314, 62.2942) -> (64.8013, 64.7942)
  line L322 (74.9615, 64.7942) -> (70.6314, 62.2942)
  line L323 (70.6314, 62.2942) -> (70.6314, 57.2942)
  line L324 (70.6314, 57.2942) -> (74.9615, 54.7942)
  line L325 (74.9615, 54.7942) -> (79.2916, 57.2942)
  line L326 (79.2916, 57.2942) -> (79.2916, 62.2942)
  line L327 (79.2916, 62.2942) -> (74.9615, 64.7942)
  line L328 (85.1218, 64.7942) -> (80.7916, 62.2942)
  line L329 (80.7916, 62.2942) -> (80.7916, 57.2942)
  line L330 (80.7916, 57.2942) -> (85.1218, 54.7942)
  line L331 (85.1218, 54.7942) -> (89.4519, 57.2942)
  line L332 (89.4519, 57.2942) -> (89.4519, 62.2942)
  line L333 (89.4519, 62.2942) -> (85.1218, 64.7942)
  line L334 (95.282, 64.7942) -> (90.9519, 62.2942)
  line L335 (90.9519, 62.2942) -> (90.9519, 57.2942)
  line L336 (90.9519, 57.2942) -> (95.282, 54.7942)
  line L337 (95.282, 54.7942) -> (99.6122, 57.2942)
  line L338 (99.6122, 57.2942) -> (99.6122, 62.2942)
  line L339 (99.6122, 62.2942) -> (95.282, 64.7942)
  line L340 (105.4423, 64.7942) -> (101.1122, 62.2942)
  line L341 (101.1122, 62.2942) -> (101.1122, 57.2942)
  line L342 (101.1122, 57.2942) -> (105.4423, 54.7942)
  line L343 (105.4423, 54.7942) -> (109.7724, 57.2942)
  line L344 (109.7724, 57.2942) -> (109.7724, 62.2942)
  line L345 (109.7724, 62.2942) -> (105.4423, 64.7942)
  line L346 (19.0801, 73.5933) -> (14.75, 71.0933)
  line L347 (14.75, 71.0933) -> (14.75, 66.0933)
  line L348 (14.75, 66.0933) -> (19.0801, 63.5933)
  line L349 (19.0801, 63.5933) -> (23.4103, 66.0933)
  line L350 (23.4103, 66.0933) -> (23.4103, 71.0933)
  line L351 (23.4103, 71.0933) -> (19.0801, 73.5933)
  line L352 (29.2404, 73.5933) -> (24.9103, 71.0933)
  line L353 (24.9103, 71.0933) -> (24.9103, 66.0933)
  line L354 (24.9103, 66.0933) -> (29.2404, 63.5933)
  line L355 (29.2404, 63.5933) -> (33.5705, 66.0933)
  line L356 (33.5705, 66.0933) -> (33.5705, 71.0933)
  line L357 (33.5705, 71.0933) -> (29.2404, 73.5933)
  line L358 (39.4006, 73.5933) -> (35.0705, 71.0933)
  line L359 (35.0705, 71.0933) -> (35.0705, 66.0933)
  line L360 (35.0705, 66.0933) -> (39.4006, 63.5933)
  line L361 (39.4006, 63.5933) -> (43.7308, 66.0933)
  line L362 (43.7308, 66.0933) -> (43.7308, 71.0933)
  line L363 (43.7308, 71.0933) -> (39.4006, 73.5933)
  line L364 (49.5609, 73.5933) -> (45.2308, 71.0933)
  line L365 (45.2308, 71.0933) -> (45.2308, 66.0933)
  line L366 (45.2308, 66.0933) -> (49.5609, 63.5933)
  line L367 (49.5609, 63.5933) -> (53.891, 66.0933)
  line L368 (53.891, 66.0933) -> (53.891, 71.0933)
  line L369 (53.891, 71.0933) -> (49.5609, 73.5933)
  line L370 (59.7211, 73.5933) -> (55.391, 71.0933)
  line L371 (55.391, 71.0933) -> (55.391, 66.0933)
  line L372 (55.391, 66.0933) -> (59.7211, 63.5933)
  line L373 (59.7211, 63.5933) -> (64.0513, 66.0933)
  line L374 (64.0513, 66.0933) -> (64.0513, 71.0933)
  line L375 (64.0513, 71.0933) -> (59.7211, 73.5933)
  line L376 (69.8814, 73.5933) -> (65.5513, 71.0933)
  line L377 (65.5513, 71.0933) -> (65.5513, 66.0933)
  line L378 (65.5513, 66.0933) -> (69.8814, 63.5933)
  line L379 (69.8814, 63.5933) -> (74.2115, 66.0933)
  line L380 (74.2115, 66.0933) -> (74.2115, 71.0933)
  line L381 (74.2115, 71.0933) -> (69.8814, 73.5933)
  line L382 (80.0416, 73.5933) -> (75.7115, 71.0933)
  line L383 (75.7115, 71.0933) -> (75.7115, 66.0933)
  line L384 (75.7115, 66.0933) -> (80.0416, 63.5933)
  line L385 (80.0416, 63.5933) -> (84.3718, 66.0933)
  line L386 (84.3718, 66.0933) -> (84.3718, 71.0933)
  line L387 (84.3718, 71.0933) -> (80.0416, 73.5933)
  line L388 (90.2019, 73.5933) -> (85.8718, 71.0933)
  line L389 (85.8718, 71.0933) -> (85.8718, 66.0933)
  line L390 (85.8718, 66.0933) -> (90.2019, 63.5933)
  line L391 (90.2019, 63.5933) -> (94.532, 66.0933)
  line L392 (94.532, 66.0933) -> (94.532, 71.0933)
  line L393 (94.532, 71.0933) -> (90.2019, 73.5933)
  line L394 (100.3622, 73.5933) -> (96.032, 71.0933)
  line L395 (96.032, 71.0933) -> (96.032, 66.0933)
  line L396 (96.032, 66.0933) -> (100.3622, 63.5933)
  line L397 (100.3622, 63.5933) -> (104.6923, 66.0933)
  line L398 (104.6923, 66.0933) -> (104.6923, 71.0933)
  line L399 (104.6923, 71.0933) -> (100.3622, 73.5933)
  line L400 (14, 82.3923) -> (9.6699, 79.8923)
  line L401 (9.6699, 79.8923) -> (9.6699, 74.8923)
  line L402 (9.6699, 74.8923) -> (14, 72.3923)
  line L403 (14, 72.3923) -> (18.3301, 74.8923)
  line L404 (18.3301, 74.8923) -> (18.3301, 79.8923)
  line L405 (18.3301, 79.8923) -> (14, 82.3923)
  line L406 (24.1603, 82.3923) -> (19.8301, 79.8923)
  line L407 (19.8301, 79.8923) -> (19.8301, 74.8923)
  line L408 (19.8301, 74.8923) -> (24.1603, 72.3923)
  line L409 (24.1603, 72.3923) -> (28.4904, 74.8923)
  line L410 (28.4904, 74.8923) -> (28.4904, 79.8923)
  line L411 (28.4904, 79.8923) -> (24.1603, 82.3923)
  line L412 (34.3205, 82.3923) -> (29.9904, 79.8923)
  line L413 (29.9904, 79.8923) -> (29.9904, 74.8923)
  line L414 (29.9904, 74.8923) -> (34.3205, 72.3923)
  line L415 (34.3205, 72.3923) -> (38.6506, 74.8923)
  line L416 (38.6506, 74.8923) -> (38.6506, 79.8923)
  line L417 (38.6506, 79.8923) -> (34.3205, 82.3923)
  line L418 (44.4808, 82.3923) -> (40.1506, 79.8923)
  line L419 (40.1506, 79.8923) -> (40.1506, 74.8923)
  line L420 (40.1506, 74.8923) -> (44.4808, 72.3923)
  line L421 (44.4808, 72.3923) -> (48.8109, 74.8923)
  line L422 (48.8109, 74.8923) -> (48.8109, 79.8923)
  line L423 (48.8109, 79.8923) -> (44.4808, 82.3923)
  line L424 (54.641, 82.3923) -> (50.3109, 79.8923)
  line L425 (50.3109, 79.8923) -> (50.3109, 74.8923)
  line L426 (50.3109, 74.8923) -> (54.641, 72.3923)
  line L427 (54.641, 72.3923) -> (58.9711, 74.8923)
  line L428 (58.9711, 74.8923) -> (58.9711, 79.8923)
  line L429 (58.9711, 79.8923) -> (54.641, 82.3923)
  line L430 (64.8013, 82.3923) -> (60.4711, 79.8923)
  line L431 (60.4711, 79.8923) -> (60.4711, 74.8923)
  line L432 (60.4711, 74.8923) -> (64.8013, 72.3923)
  line L433 (64.8013, 72.3923) -> (69.1314, 74.8923)
  line L434 (69.1314, 74.8923) -> (69.1314, 79.8923)
  line L435 (69.1314, 79.8923) -> (64.8013, 82.3923)
  line L436 (74.9615, 82.3923) -> (70.6314, 79.8923)
  line L437 (70.6314, 79.8923) -> (70.6314, 74.8923)
  line L438 (70.6314, 74.8923) -> (74.9615, 72.3923)
  line L439 (74.9615, 72.3923) -> (79.2916, 74.8923)
  line L440 (79.2916, 74.8923) -> (79.2916, 79.8923)
  line L441 (79.2916, 79.8923) -> (74.9615, 82.3923)
  line L442 (85.1218, 82.3923) -> (80.7916, 79.8923)
  line L443 (80.7916, 79.8923) -> (80.7916, 74.8923)
  line L444 (80.7916, 74.8923) -> (85.1218, 72.3923)
  line L445 (85.1218, 72.3923) -> (89.4519, 74.8923)
  line L446 (89.4519, 74.8923) -> (89.4519, 79.8923)
  line L447 (89.4519, 79.8923) -> (85.1218, 82.3923)
  line L448 (95.282, 82.3923) -> (90.9519, 79.8923)
  line L449 (90.9519, 79.8923) -> (90.9519, 74.8923)
  line L450 (90.9519, 74.8923) -> (95.282, 72.3923)
  line L451 (95.282, 72.3923) -> (99.6122, 74.8923)
  line L452 (99.6122, 74.8923) -> (99.6122, 79.8923)
  line L453 (99.6122, 79.8923) -> (95.282, 82.3923)
  line L454 (105.4423, 82.3923) -> (101.1122, 79.8923)
  line L455 (101.1122, 79.8923) -> (101.1122, 74.8923)
  line L456 (101.1122, 74.8923) -> (105.4423, 72.3923)
  line L457 (105.4423, 72.3923) -> (109.7724, 74.8923)
  line L458 (109.7724, 74.8923) -> (109.7724, 79.8923)
  line L459 (109.7724, 79.8923) -> (105.4423, 82.3923)
  line L460 (19.0801, 91.1913) -> (14.75, 88.6913)
  line L461 (14.75, 88.6913) -> (14.75, 83.6913)
  line L462 (14.75, 83.6913) -> (19.0801, 81.1913)
  line L463 (19.0801, 81.1913) -> (23.4103, 83.6913)
  line L464 (23.4103, 83.6913) -> (23.4103, 88.6913)
  line L465 (23.4103, 88.6913) -> (19.0801, 91.1913)
  line L466 (29.2404, 91.1913) -> (24.9103, 88.6913)
  line L467 (24.9103, 88.6913) -> (24.9103, 83.6913)
  line L468 (24.9103, 83.6913) -> (29.2404, 81.1913)
  line L469 (29.2404, 81.1913) -> (33.5705, 83.6913)
  line L470 (33.5705, 83.6913) -> (33.5705, 88.6913)
  line L471 (33.5705, 88.6913) -> (29.2404, 91.1913)
  line L472 (39.4006, 91.1913) -> (35.0705, 88.6913)
  line L473 (35.0705, 88.6913) -> (35.0705, 83.6913)
  line L474 (35.0705, 83.6913) -> (39.4006, 81.1913)
  line L475 (39.4006, 81.1913) -> (43.7308, 83.6913)
  line L476 (43.7308, 83.6913) -> (43.7308, 88.6913)
  line L477 (43.7308, 88.6913) -> (39.4006, 91.1913)
  line L478 (49.5609, 91.1913) -> (45.2308, 88.6913)
  line L479 (45.2308, 88.6913) -> (45.2308, 83.6913)
  line L480 (45.2308, 83.6913) -> (49.5609, 81.1913)
  line L481 (49.5609, 81.1913) -> (53.891, 83.6913)
  line L482 (53.891, 83.6913) -> (53.891, 88.6913)
  line L483 (53.891, 88.6913) -> (49.5609, 91.1913)
  line L484 (59.7211, 91.1913) -> (55.391, 88.6913)
  line L485 (55.391, 88.6913) -> (55.391, 83.6913)
  line L486 (55.391, 83.6913) -> (59.7211, 81.1913)
  line L487 (59.7211, 81.1913) -> (64.0513, 83.6913)
  line L488 (64.0513, 83.6913) -> (64.0513, 88.6913)
  line L489 (64.0513, 88.6913) -> (59.7211, 91.1913)
  line L490 (69.8814, 91.1913) -> (65.5513, 88.6913)
  line L491 (65.5513, 88.6913) -> (65.5513, 83.6913)
  line L492 (65.5513, 83.6913) -> (69.8814, 81.1913)
  line L493 (69.8814, 81.1913) -> (74.2115, 83.6913)
  line L494 (74.2115, 83.6913) -> (74.2115, 88.6913)
  line L495 (74.2115, 88.6913) -> (69.8814, 91.1913)
  line L496 (80.0416, 91.1913) -> (75.7115, 88.6913)
  line L497 (75.7115, 88.6913) -> (75.7115, 83.6913)
  line L498 (75.7115, 83.6913) -> (80.0416, 81.1913)
  line L499 (80.0416, 81.1913) -> (84.3718, 83.6913)
  line L500 (84.3718, 83.6913) -> (84.3718, 88.6913)
  line L501 (84.3718, 88.6913) -> (80.0416, 91.1913)
  line L502 (90.2019, 91.1913) -> (85.8718, 88.6913)
  line L503 (85.8718, 88.6913) -> (85.8718, 83.6913)
  line L504 (85.8718, 83.6913) -> (90.2019, 81.1913)
  line L505 (90.2019, 81.1913) -> (94.532, 83.6913)
  line L506 (94.532, 83.6913) -> (94.532, 88.6913)